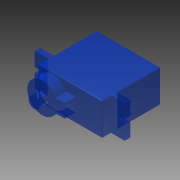
# Autodesk Inventor part: Servo Motor
Saved by Autodesk Inventor 2013 (Build 170138000, 138)
## iProperties
Created: 2012-10-28
Part Number: Servo Motor
Material: Generic
Document SubType Name: Modeling
Designer: uqgtayle
Density: 1 g/cm^3
Author: uqgtayle
Autodesk Inventor part; units mm, degrees
ref_plane "YZ Plane" through (0, 0, 0) normal (1, 0, 0) x (0, 1, 0)
ref_plane "XZ Plane" through (0, 0, 0) normal (0, 1, 0) x (-1, 0, 0)
ref_plane "XY Plane" through (0, 0, 0) normal (0, 0, 1) x (1, 0, 0)
sketch "Sketch1" plane through (0, 0, 0) normal (0, 0, 1) x (1, 0, 0)
  line L0 (0, 0) -> (23.5, 0)
  line L1 (23.5, 0) -> (23.5, -21.5)
  line L2 (23.5, -21.5) -> (0, -21.5)
  line L3 (0, -21.5) -> (0, 0)
  dimension "d0" = 23.5
  dimension "d1" = 21.5
  constraints: 8 end point, 2 parallel, 1 horizontal, 1 perpendicular
  measures "d0" distance of L0.start L0.end
  measures "d1" distance of L2.end L0.start
extrude "Extrusion1" add sketch "Sketch1" against normal blind 12
sketch "Sketch2" plane through (0, 0, 0) normal (0, 0, 1) x (1, 0, 0)
  line L0 (0, 0) -> (23.5, 0) projected
  line L1 (0, -21.5) -> (0, 0) projected
  line L2 (23.5, 0) -> (23.5, -21.5) projected
  line L3 (-4.75, -16) -> (28.25, -16)
  line L4 (28.25, -16) -> (28.25, -18)
  line L5 (28.25, -18) -> (-4.75, -18)
  line L6 (-4.75, -18) -> (-4.75, -16)
  dimension "d4" = 16
  dimension "d5" = 4.75
  dimension "d6" = 4.75
  dimension "d7" = 2
  constraints: 8 end point, 2 parallel, 1 horizontal, 1 perpendicular
  measures "d4" distance between parallel lines of L3 L0
  measures "d5" distance between parallel lines of L6 L1
  measures "d6" distance between parallel lines of L4 L2
  measures "d7" distance of L3.end L4.end
extrude "Extrusion2" add sketch "Sketch2" against normal blind 12 contours L3 L2 L5 L1 | L1 L5 L6 L3 | L3 L4 L5 L2
sketch "Sketch3" plane through (0, -21.5, 0) normal (0, -1, 0) x (1, 0, 0)
  line L0 (0, 0) -> (0, -12) projected
  circle A0 centre (5.5, -6) radius 5.5
  dimension "d10" = 5.5
  dimension "d11" = 11
  constraints: 1 centre point
  measures "d10" distance from line of L0 A0.centre
  measures "d11" diameter of A0
extrude "Extrusion3" add sketch "Sketch3" along normal blind 4
sketch "Sketch4" plane through (5.5, -25.5, -6) normal (0, -1, 0) x (1, 0, 0)
  circle A0 centre (0, 0) radius 5.5 projected
  line L0 (4.8288, 2.5) -> (8.25, 2.5)
  line L1 (8.25, 2.5) -> (8.25, -2.5)
  line L2 (8.25, -2.5) -> (4.8288, -2.5)
  line L3 (4.8288, -2.5) -> (4.8288, 2.5)
  point P0 (-5.5, 6)
  point P1 (8.25, 0)
  dimension "d15" = 5
  dimension "d17" = 8.25
  constraints: 8 end point, 2 parallel, 1 horizontal, 1 horizontal alignment, 1 midpoint, 1 perpendicular
  measures "d15" distance of L0.end L1.end
  measures "d17" distance of point (8.25, 0) A0.centre
extrude "Extrusion4" add sketch "Sketch4" against normal blind 4 contours A0 L2 L3 L0 | A0 L0 L1 L2 picked at (4.9626, -0.5673)
sketch "Sketch5" plane through (0, -25.5, 0) normal (0, -1, 0) x (1, 0, 0)
  arc A0 (10.399, -3.5) -> (10.399, -8.5) centre (5.5, -6) ccw projected
  circle A1 centre (5.5, -6) radius 2
  point P0 (0, 0)
  dimension "d20" = 4
  constraints: 1 centre point, 1 coincident
  measures "d20" diameter of A1
extrude "Extrusion5" add sketch "Sketch5" along normal blind 3
sketch "Sketch6" plane through (-4.75, -18, 0) normal (0, -1, 0) x (1, 0, 0)
  line L0 (4.75, 0) -> (4.75, -12) projected
  line L1 (0, 0) -> (0, -12) projected
  line L2 (28.25, -12) -> (28.25, 0) projected
  line L3 (33, -12) -> (28.25, -12) projected
  line L4 (33, 0) -> (33, -12) projected
  line L5 (33, 0) -> (28.25, 0) projected
  circle A0 centre (2, -6) radius 1.1
  circle A1 centre (31, -6) radius 1.1
  line L6 (-3.3152, -5.1) -> (1.5271, -5.1)
  line L7 (1.5271, -5.1) -> (1.5271, -6.9)
  line L8 (1.5271, -6.9) -> (-3.3152, -6.9)
  line L9 (-3.3152, -6.9) -> (-3.3152, -5.1)
  line L10 (31.5226, -5.1) -> (37.6277, -5.1)
  line L11 (37.6277, -5.1) -> (37.6277, -6.9)
  line L12 (37.6277, -6.9) -> (31.5226, -6.9)
  line L13 (31.5226, -6.9) -> (31.5226, -5.1)
  point P0 (4.75, -6)
  point P1 (1.5271, -6)
  point P2 (28.25, -6)
  point P3 (31.5226, -6)
  dimension "d24" = 2.2
  dimension "d26" = 2
  dimension "d27" = 2
  dimension "d28" = 2.2
  dimension "d29" = 1.8
  dimension "d30" = 1.8
  constraints: 16 end point, 4 horizontal alignment, 4 midpoint, 4 parallel, 2 centre point, 2 horizontal, 2 perpendicular
  measures "d24" diameter of A0
  measures "d26" distance from line of L4 A1.centre
  measures "d27" distance from line of A0.centre L1
  measures "d28" diameter of A1
  measures "d29" distance of L10.end L11.end
  measures "d30" distance of L8.end L6.start
extrude "Extrusion6" cut sketch "Sketch6" against normal through all contours L6 A0 L8 L1 | L1 L8 L9 L6 | L6 L7 L8 A0 | A0 L8 L7 L6 | L12 A1 L10 L4 | L4 L10 L11 L12 | L12 L13 L10 A1 | A1 L10 L13 L12
fillet "Fillet1" radius 0.5 13 edges at (0, -8, -12) (23.5, -8, -12) (11.75, 0, -12) (11.75, 0, 0) (0, 0, -6) (23.5, 0, -6) (0, -8, 0) (23.5, -8, 0) (23.5, -19.75, 0) (23.5, -21.5, -6) (23.5, -19.75, -12) (11.75, -21.5, -12) (11.75, -21.5, 0)
equation "\"d6\" = d5"
body "Solid1"
